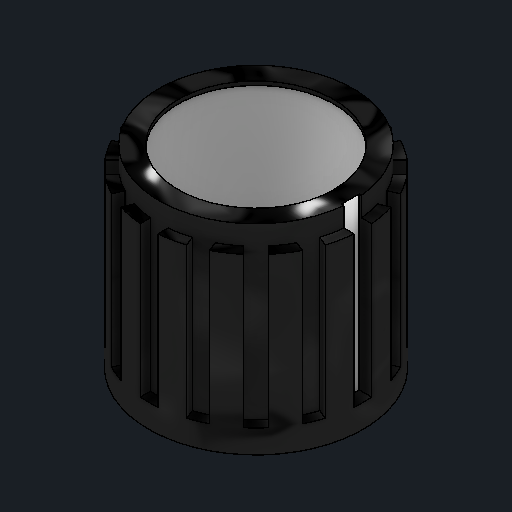
# Autodesk Inventor part: Knob3
Saved by Autodesk Inventor 2026.2 (Build 302298000, 298)
## iProperties
Created: 2015-05-06
Part Number: Knob3
Material: Generic
Document SubType Name: Modeling
Designer: Philip
Density: 1 g/cm^3
Appearance: Black
Author: Philip
Autodesk Inventor part; units mm, degrees
ref_plane "YZ Plane" through (0, 0, 0) normal (1, 0, 0) x (0, 1, 0)
ref_plane "XZ Plane" through (0, 0, 0) normal (0, 1, 0) x (-1, 0, 0)
ref_plane "XY Plane" through (0, 0, 0) normal (0, 0, 1) x (1, 0, 0)
sketch "Sketch1" plane through (0, 0, 0) normal (0, 1, 0) x (-1, 0, 0)
  circle A0 centre (0, 0) radius 6.985
  dimension "d0" = 13.97
  constraints: 1 centre point, 1 coincident
  measures "d0" diameter of A0
extrude "Extrusion1" add sketch "Sketch1" along normal blind 12.573
sketch "Sketch2" plane through (0, 12.573, 0) normal (0, 1, 0) x (1, 0, 0)
  circle A0 centre (0, 0) radius 6.3246
  circle A1 centre (0, 0) radius 6.985 projected
  dimension "d3" = 12.6492
  constraints: 1 centre point, 1 coincident
  measures "d3" diameter of A0
extrude "Extrusion2" cut sketch "Sketch2" against normal blind 1.27
sketch "Sketch3" plane through (0, 11.303, 0) normal (0, 1, 0) x (1, 0, 0)
  circle A0 centre (0, 0) radius 6.3246 projected
  circle A1 centre (0, 0) radius 6.985 projected
  circle A2 centre (0, 0) radius 6.985 projected
  line L0 (-6.9616, -0.5715) -> (-6.2987, -0.5715)
  line L1 (-6.9616, 0.5715) -> (-6.2987, 0.5715)
  dimension "d6" = 1.143
  dimension "d7" = 0.5715
  constraints: 6 point on circle, 4 end point, 2 horizontal
  measures "d6" distance between parallel lines of L1 L0
  measures "d7" distance from line of L1 point (0, 0)
extrude "Extrusion3" cut sketch "Sketch3" against normal blind 9.779 contours A0 L0 A1 L1 picked at (-6.5273, 0.4446)
pattern_circular "Circular Pattern1" count 16 over 360 about axis through (0, 0, 0) along (0, 1, 0) of "Extrusion3"
sketch "Sketch4" plane through (0, 12.573, 0) normal (0, 1, 0) x (1, 0, 0)
  circle A0 centre (0, 0) radius 5.08
  dimension "d13" = 10.16
  constraints: 1 centre point, 1 coincident
  measures "d13" diameter of A0
extrude "Extrusion4" cut sketch "Sketch4" against normal blind 0.254
sketch "Sketch5" plane through (0, 12.573, 0) normal (0, 1, 0) x (1, 0, 0)
  line L0 (6.2987, 0.5715) -> (6.9616, 0.5715) projected
  line L1 (6.9616, -0.5715) -> (6.2987, -0.5715) projected
  circle A0 centre (0, 0) radius 6.3246 projected
  line L2 (6.2987, 0.5715) -> (6.1474, 0.5715)
  line L3 (6.1474, 0.5715) -> (6.1474, -0.5715)
  line L4 (6.1474, -0.5715) -> (6.2987, -0.5715)
  constraints: 6 end point, 2 perpendicular, 1 horizontal
extrude "Extrusion5" cut sketch "Sketch5" against normal blind 11.049 contours A0 L4 L3 L2 picked at (6.2065, 0)
equation "\"d7\" = 0.5 * d6"
body "Solid1"
